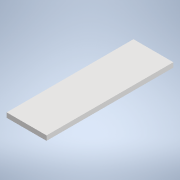
# Autodesk Inventor part: housing_bottom
Saved by Autodesk Inventor 2022 (Build 260153000, 153)
## iProperties
Created: 2023-03-07
Part Number: housing_bottom
Material: Generic
Document SubType Name: Modeling
Designer: galad
Density: 1 g/cm^3
Appearance: Default
Author: galad
Autodesk Inventor part; units mm, degrees
ref_plane "YZ Plane" through (0, 0, 0) normal (1, 0, 0) x (0, 1, 0)
ref_plane "XZ Plane" through (0, 0, 0) normal (0, 1, 0) x (-1, 0, 0)
ref_plane "XY Plane" through (0, 0, 0) normal (0, 0, 1) x (1, 0, 0)
sketch "Sketch1" plane through (0, 0, 0) normal (0, 1, 0) x (-1, 0, 0)
  line L0 (24.7933, -42.1134) -> (-6.7642, -42.1134)
  line L1 (-6.7642, -42.1134) -> (-6.7642, 45.097)
  line L2 (-6.7642, 45.097) -> (24.7933, 45.097)
  line L3 (24.7933, 45.097) -> (24.7933, -42.1134)
  line L4 (21.7933, -39.1134) -> (-3.7642, -39.1134)
  line L5 (-3.7642, -39.1134) -> (-3.7642, 42.097)
  line L6 (-3.7642, 42.097) -> (21.7933, 42.097)
  line L7 (21.7933, 42.097) -> (21.7933, -39.1134)
  point P0 (0, 0)
  dimension "d0" = 3
  dimension "d1" = 3
  dimension "d2" = 3
  dimension "d3" = 3
  constraints: 16 end point, 4 parallel, 2 horizontal, 2 perpendicular
  measures "d0" distance between parallel lines of L4 L0
  measures "d1" distance between parallel lines of L1 L5
  measures "d2" distance between parallel lines of L3 L7
  measures "d3" distance between parallel lines of L2 L6
extrude "Extrusion2" add sketch "Sketch1" against normal blind 3 contours L0 L1 L2 L3 | L4 L5 L6 L7
extrude "Extrusion3" add sketch "Sketch1" along normal blind 10
body "Solid2"
